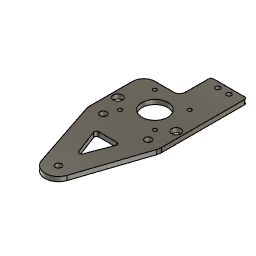
Laser Carriage - Motor Side V2 (Autodesk Fusion 360 design; units mm, degrees)
Autodesk Fusion 360 part; units mm, degrees
sketch "Sketch1" plane through (0, 0, 0) normal (0, 0, 1) x (1, 0, 0) in component "Laser Carriage - Motor Side V2"
  line L0 (0, 0) -> (64, 0)
  line L1 (64, 0) -> (64, 120)
  line L2 (64, 120) -> (0, 120)
  line L3 (0, 120) -> (0, 0)
  dimension "d1" = 64
  dimension "d2" = 120
  constraint horizontal L0
  constraint vertical L1
  constraint horizontal L2
  constraint vertical L3
  constraint coincident L0.start L3.end
  measures "d1" distance of L0.start L0.end
  measures "d2" distance of L0.start L2.end
extrude "Extrude1" add sketch "Sketch1" along normal blind 4 in component "Laser Carriage - Motor Side V2"
sketch "Sketch2" plane through (0, 0, 4) normal (0, 0, 1) x (-1, 0, 0) in component "Laser Carriage - Motor Side V2"
  line L0 (0, -120) -> (0, 0)
  line L1 (0, 0) -> (-64, 0)
  line L2 (-64, 0) -> (-64, -120)
  line L3 (-64, -120) -> (0, -120)
  line L4 (-12, -120) -> (-12, 0) construction
  line L5 (-52, -120) -> (-52, 0) construction
  line L6 (0, -12) -> (-64, -12) construction
  line L7 (0, -72) -> (-64, -72) construction
  circle A0 centre (-12, -72) radius 12 construction
  circle A1 centre (-52, -72) radius 12 construction
  circle A2 centre (-12, -72) radius 3
  circle A3 centre (-52, -72) radius 3
  circle A4 centre (-32, -12) radius 12 construction
  circle A5 centre (-32, -12) radius 2.75
  line L8 (0, -85) -> (-64, -85) construction
  line L9 (-32, -85) -> (-32, 0) construction
  line L10 (0, -42) -> (-64, -42) construction
  line L11 (0, -27) -> (-64, -27) construction
  line L12 (0, -56) -> (-64, -56) construction
  line L13 (-21, -56) -> (-21, -27) construction
  line L14 (-43, -56) -> (-43, -27) construction
  line L15 (-21, -56) -> (-43, -56)
  line L16 (-43, -56) -> (-32, -27)
  line L17 (-32, -27) -> (-21, -56)
  point P0 (-32, -42)
  dimension "d8" = 12
  dimension "d13" = 24
  dimension "d14" = 24
  dimension "d16" = 6
  dimension "d17" = 6
  dimension "d40" = 60
  dimension "d53" = 24
  dimension "d55" = 5.5
  dimension "d234" = 13
  dimension "d238" = 20
  dimension "d324" = 30
  dimension "d327" = 20
  dimension "d333" = 15
  dimension "d334" = 56
  dimension "d335" = 11
  dimension "d336" = 11
  constraint coincident L3 L4.start
  constraint coincident L1 L4.end
  constraint perpendicular L1 L4
  constraint coincident L3 L5.start
  constraint coincident L1 L5.end
  constraint perpendicular L1 L5
  constraint coincident L1 L9.end
  constraint coincident L0 L6.start
  constraint coincident L2 L6.end
  constraint perpendicular L2 L6
  constraint coincident L0 L7.start
  constraint coincident L2 L7.end
  constraint perpendicular L2 L7
  constraint coincident L7 A0.centre
  constraint coincident L4 A0.centre
  constraint coincident L7 A1.centre
  constraint coincident L5 A1.centre
  constraint concentric A0 A2
  constraint concentric A1 A3
  constraint coincident L6 A4.centre
  constraint concentric A4 A5
  constraint coincident L0 L8.start
  constraint coincident L2 L8.end
  constraint perpendicular L2 L8
  constraint midpoint L8 L9.start
  constraint coincident L0 L10.start
  constraint coincident L2 L10.end
  constraint perpendicular L2 L10
  constraint midpoint L10 P0
  constraint coincident A4.centre L9
  constraint coincident L0 L11.start
  constraint coincident L2 L11.end
  constraint perpendicular L2 L11
  constraint coincident L0 L12.start
  constraint coincident L2 L12.end
  constraint perpendicular L2 L12
  constraint coincident L12 L13.start
  constraint coincident L11 L13.end
  constraint perpendicular L11 L13
  constraint coincident L11 L14.end
  constraint perpendicular L11 L14
  constraint midpoint L11 L16.end
  constraint coincident L12 L14.start
  measures "d8" distance of L1 L6
  measures "d13" diameter of A0
  measures "d14" diameter of A1
  measures "d16" diameter of A2
  measures "d17" diameter of A3
  measures "d40" distance of L6 L7
  measures "d53" diameter of A4
  measures "d55" diameter of A5
  measures "d234" distance of A0.centre L8
  measures "d238" distance of L4 L9
  measures "d324" distance of L6 L10
  measures "d327" distance of L5 L9
  measures "d333" distance of L6 L11
  measures "d334" distance of L1 L12
  measures "d335" distance of L9 L13
  measures "d336" distance of L9 L14
extrude "Extrude2" cut sketch "Sketch2" against normal up to surface (4 mm away) contours A2 | A3 | A5 | L15 L16 L17 in component "Laser Carriage - Motor Side V2"
sketch "Sketch16" plane through (0, 0, 4) normal (0, 0, 1) x (-1, 0, 0) in component "Laser Carriage - Motor Side V2"
  circle A0 centre (-52, -72) radius 3
  circle A1 centre (-12, -72) radius 3
  line L0 (-64, -120) -> (0, -120)
  line L1 (0, -120) -> (0, 0)
  line L2 (0, 0) -> (-64, 0)
  line L3 (-64, 0) -> (-64, -120)
  circle A2 centre (-32, -12) radius 2.75
  line L4 (0, -91) -> (-64, -91) construction
  line L5 (-64, -120) -> (0, -120) construction
  line L6 (-6, 0) -> (-6, -120) construction
  line L7 (0, -120) -> (0, 0) construction
  line L8 (-58, 0) -> (-58, -120) construction
  circle A3 centre (-6, -91) radius 4
  circle A4 centre (-58, -91) radius 4
  line L9 (0, 0) -> (-64, 0)
  line L10 (-43, -56) -> (-32, -27)
  line L11 (-32, -27) -> (-21, -56)
  line L12 (-21, -56) -> (-43, -56)
  dimension "d268" = 6
  dimension "d269" = 6
  dimension "d270" = 8
  dimension "d271" = 8
  dimension "d273" = 91
  constraint coincident L1 L4.start
  constraint coincident L3 L4.end
  constraint perpendicular L3 L4
  constraint coincident L5 L6.end
  constraint coincident L2 L8.start
  constraint coincident L5 L8.end
  constraint coincident L4 A3.centre
  constraint coincident L6 A3.centre
  constraint coincident L4 A4.centre
  constraint coincident L8 A4.centre
  measures "d268" distance of L6 L7
  measures "d269" distance of L3 L8
  measures "d270" diameter of A3
  measures "d271" diameter of A4
  measures "d273" distance of L2 L4
extrude "Extrude17" cut sketch "Sketch16" against normal up to surface (4 mm away) contours A3 | A4 in component "Laser Carriage - Motor Side V2"
sketch "Sketch18" plane through (0, 0, 4) normal (0, 0, 1) x (-1, 0, 0) in component "Laser Carriage - Motor Side V2"
  line L0 (-64, -120) -> (0, -120)
  line L1 (-32, -120) -> (-32, 0) construction
  line L2 (0, 0) -> (-64, 0) construction
  line L3 (-47.5, -120) -> (-47.5, 0) construction
  line L4 (-16.5, 0) -> (-16.5, -120) construction
  line L5 (-2, -113.5) -> (-62, -113.5) construction
  line L6 (-2, -82.5) -> (-62, -82.5) construction
  line L7 (-2, -98) -> (-62, -98) construction
  circle A0 centre (-32, -98) radius 11.5
  circle A1 centre (-16.5, -113.5) radius 1.65
  circle A2 centre (-47.5, -113.5) radius 1.65
  circle A3 centre (-16.5, -82.5) radius 1.65
  circle A4 centre (-47.5, -82.5) radius 1.65
  line L8 (-2, -120) -> (-62, -120) construction
  line L9 (-54, -120) -> (-10, -120) construction
  line L10 (-10, -120) -> (-10, -76) construction
  line L11 (-10, -76) -> (-54, -76) construction
  line L12 (-54, -76) -> (-54, -120) construction
  line L13 (-54, -120) -> (-10, -76) construction
  line L14 (-10, -120) -> (-54, -76) construction
  point P0 (-32, -98)
  dimension "d275" = 15.5
  dimension "d276" = 15.5
  dimension "d279" = 98
  dimension "d280" = 15.5
  dimension "d281" = 15.5
  dimension "d283" = 23
  dimension "d284" = 3.3
  dimension "d285" = 3.3
  dimension "d286" = 3.3
  dimension "d287" = 3.3
  dimension "d288" = 6.5
  dimension "d289" = 44
  dimension "d290" = 44
  constraint midpoint L0 L1.start
  constraint perpendicular L0 L1
  constraint coincident L0 L3.start
  constraint coincident L2 L3.end
  constraint perpendicular L2 L3
  constraint coincident L2 L4.start
  constraint coincident L0 L4.end
  constraint perpendicular L0 L4
  constraint horizontal L5
  constraint horizontal L6
  constraint perpendicular L3 L7
  constraint midpoint L7 P0
  constraint coincident L4 A1.centre
  constraint coincident L5 A1.centre
  constraint coincident L3 A2.centre
  constraint coincident L5 A2.centre
  constraint coincident L4 A3.centre
  constraint coincident L6 A3.centre
  constraint coincident L3 A4.centre
  constraint coincident L6 A4.centre
  constraint perpendicular L3 L8
  constraint horizontal L9
  constraint perpendicular L9 L10
  constraint parallel L9 L11
  constraint parallel L10 L12
  constraint coincident L13 P0
  constraint coincident L14 P0
  constraint coincident P0 A0.centre
  measures "d275" distance of L1 L3
  measures "d276" distance of L1 L4
  measures "d279" distance of L2 L7
  measures "d280" distance of L5 L7
  measures "d281" distance of L6 L7
  measures "d283" diameter of A0
  measures "d284" diameter of A1
  measures "d285" diameter of A2
  measures "d286" diameter of A3
  measures "d287" diameter of A4
  measures "d288" distance of L5 L8
  measures "d289" distance of L10.end L11.end
  measures "d290" distance of L9.end L10.end
extrude "Extrude18" cut sketch "Sketch18" against normal up to surface (4 mm away) in component "Laser Carriage - Motor Side V2"
sketch "Sketch20" plane through (0, 0, 0) normal (0, 0, -1) x (1, 0, 0) in component "Laser Carriage - Motor Side V2"
  circle A0 centre (16.5, -113.5) radius 1.65
  circle A1 centre (47.5, -113.5) radius 1.65
  circle A2 centre (16.5, -82.5) radius 1.65
  circle A3 centre (32, -98) radius 11.5
  circle A4 centre (47.5, -82.5) radius 1.65
  circle A5 centre (6, -91) radius 4
  circle A6 centre (58, -91) radius 4
  circle A7 centre (52, -72) radius 3
  circle A8 centre (32, -12) radius 2.75
  circle A9 centre (12, -72) radius 3
  line L0 (0, 0) -> (0, -120)
  line L1 (0, -120) -> (64, -120)
  line L2 (64, -120) -> (64, 0)
  line L3 (64, 0) -> (0, 0)
  line L4 (64, -120) -> (64, -148)
  line L5 (32, -120) -> (32, -148)
  line L6 (32, -148) -> (64, -148)
  line L7 (32, -27) -> (43, -56)
  line L8 (43, -56) -> (21, -56)
  line L9 (21, -56) -> (32, -27)
  dimension "d303" = 28
  dimension "d304" = 28
  constraint coincident L1.end L2.start
  constraint perpendicular L1 L4
  constraint midpoint L1 L5.start
  constraint perpendicular L1 L5
  measures "d303" distance of L1.end L4.end
  measures "d304" distance of L5.start L5.end
extrude "Extrude20" add sketch "Sketch20" against normal blind 4 contours L1 L4 L5 L6 in component "Laser Carriage - Motor Side V2"
sketch "Sketch21" plane through (0, 0, 4) normal (0, 0, 1) x (-1, 0, 0) in component "Laser Carriage - Motor Side V2"
  circle A0 centre (-16.5, -113.5) radius 1.65
  circle A1 centre (-47.5, -113.5) radius 1.65
  circle A2 centre (-16.5, -82.5) radius 1.65
  circle A3 centre (-32, -98) radius 11.5
  circle A4 centre (-47.5, -82.5) radius 1.65
  circle A5 centre (-6, -91) radius 4
  circle A6 centre (-58, -91) radius 4
  line L0 (0, -120) -> (0, 0)
  line L1 (0, 0) -> (-64, 0)
  line L2 (-64, 0) -> (-64, -148)
  line L3 (-64, -148) -> (-32, -148)
  line L4 (-32, -148) -> (-32, -120)
  line L5 (-32, -120) -> (0, -120)
  circle A7 centre (-52, -72) radius 3
  circle A8 centre (-32, -12) radius 2.75
  circle A9 centre (-12, -72) radius 3
  line L6 (-48, -148) -> (-48, -122) construction
  line L7 (-32, -138) -> (-64, -138) construction
  line L8 (-54, -120) -> (-10, -120) construction
  line L9 (-32, -143) -> (-64, -143) construction
  line L10 (-53, -148) -> (-53, -138) construction
  line L11 (-43, -148) -> (-43, -138) construction
  circle A10 centre (-43, -143) radius 2.05
  circle A11 centre (-53, -143) radius 2.05
  line L12 (-43, -56) -> (-32, -27)
  line L13 (-32, -27) -> (-21, -56)
  line L14 (-21, -56) -> (-43, -56)
  dimension "d309" = 18
  dimension "d310" = 5
  dimension "d311" = 10
  dimension "d312" = 5
  dimension "d313" = 4.1
  dimension "d314" = 4.1
  constraint midpoint L3 L6.start
  constraint perpendicular L3 L6
  constraint coincident L4 L7.start
  constraint coincident L2 L7.end
  constraint perpendicular L2 L7
  constraint coincident L4 L9.start
  constraint coincident L2 L9.end
  constraint perpendicular L2 L9
  constraint coincident L3 L10.start
  constraint coincident L7 L10.end
  constraint perpendicular L7 L10
  constraint coincident L3 L11.start
  constraint coincident L7 L11.end
  constraint perpendicular L7 L11
  constraint midpoint L11 A10.centre
  constraint midpoint L10 A11.centre
  measures "d309" distance of L7 L8
  measures "d310" distance of L3 L9
  measures "d311" distance of L10 L11
  measures "d312" distance of L6 L11
  measures "d313" diameter of A10
  measures "d314" diameter of A11
extrude "Extrude21" cut sketch "Sketch21" against normal blind 4 contours A10 | A11 in component "Laser Carriage - Motor Side V2"
sketch "Sketch22" plane through (0, 0, 4) normal (0, 0, 1) x (-1, 0, 0) in component "Laser Carriage - Motor Side V2"
  circle A0 centre (-43, -143) radius 2.05
  circle A1 centre (-53, -143) radius 2.05
  circle A2 centre (-16.5, -113.5) radius 1.65
  circle A3 centre (-47.5, -113.5) radius 1.65
  circle A4 centre (-16.5, -82.5) radius 1.65
  circle A5 centre (-32, -98) radius 11.5
  circle A6 centre (-47.5, -82.5) radius 1.65
  circle A7 centre (-6, -91) radius 4
  circle A8 centre (-58, -91) radius 4
  circle A9 centre (-12, -72) radius 3
  circle A10 centre (-52, -72) radius 3
  circle A11 centre (-32, -12) radius 2.75
  line L0 (0, -120) -> (0, 0)
  line L1 (0, 0) -> (-64, 0)
  line L2 (-64, 0) -> (-64, -148)
  line L3 (-64, -148) -> (-32, -148)
  line L4 (-32, -148) -> (-32, -120)
  line L5 (-32, -120) -> (0, -120)
  circle A12 centre (-12, -72) radius 12
  circle A13 centre (-52, -72) radius 12
  circle A14 centre (-32, -12) radius 12
  line L6 (-0.6158, -68.2053) -> (-20.6158, -8.2053)
  line L7 (-63.3842, -68.2053) -> (-43.3842, -8.2053)
  line L8 (-43, -56) -> (-32, -27)
  line L9 (-32, -27) -> (-21, -56)
  line L10 (-21, -56) -> (-43, -56)
  dimension "d328" = 24
  dimension "d329" = 24
  dimension "d330" = 24
  constraint concentric A9 A12
  constraint concentric A10 A13
  constraint concentric A11 A14
  constraint tangent A12 L6
  constraint tangent A14 L6
  constraint tangent A13 L7
  constraint tangent A14 L7
  constraint coincident A13 L7.start
  constraint coincident A14 L7.end
  constraint coincident A14 L6.end
  constraint coincident A12 L6.start
  measures "d328" diameter of A12
  measures "d329" diameter of A13
  measures "d330" diameter of A14
extrude "Extrude22" cut sketch "Sketch22" against normal up to surface (4 mm away) contours L0 L1 A12 A14 L6 | L1 L2 A13 A14 L7 in component "Laser Carriage - Motor Side V2"
sketch "Sketch23" plane through (0, 0, 4) normal (0, 0, 1) x (-1, 0, 0) in component "Laser Carriage - Motor Side V2"
  arc A0 (-63.3842, -68.2053) -> (-64, -72) centre (-52, -72) ccw
  line L0 (-64, -72) -> (-64, -148)
  line L1 (-64, -148) -> (-32, -148)
  line L2 (-32, -148) -> (-32, -120)
  line L3 (-32, -120) -> (0, -120)
  line L4 (0, -120) -> (0, -72)
  arc A1 (0, -72) -> (-0.6158, -68.2053) centre (-12, -72) ccw
  line L5 (-0.6158, -68.2053) -> (-20.6158, -8.2053)
  arc A2 (-20.6158, -8.2053) -> (-43.3842, -8.2053) centre (-32, -12) ccw
  line L6 (-43.3842, -8.2053) -> (-63.3842, -68.2053)
  circle A3 centre (-43, -143) radius 2.05
  circle A4 centre (-53, -143) radius 2.05
  circle A5 centre (-16.5, -113.5) radius 1.65
  circle A6 centre (-47.5, -113.5) radius 1.65
  circle A7 centre (-16.5, -82.5) radius 1.65
  circle A8 centre (-32, -98) radius 11.5
  circle A9 centre (-47.5, -82.5) radius 1.65
  circle A10 centre (-6, -91) radius 4
  circle A11 centre (-58, -91) radius 4
  circle A12 centre (-12, -72) radius 3
  circle A13 centre (-52, -72) radius 3
  circle A14 centre (-32, -12) radius 2.75
  line L7 (-43, -56) -> (-32, -27)
  line L8 (-32, -27) -> (-21, -56)
  line L9 (-21, -56) -> (-43, -56)
fillet "Fillet11" radius 5 1 edges at (32, 120, 2) in component "Laser Carriage - Motor Side V2"
fillet "Fillet11" radius 2 2 edges at (32, 148, 2) (64, 148, 2) in component "Laser Carriage - Motor Side V2"
fillet "Fillet11" radius 2 3 edges at (21, 56, 2) (43, 56, 2) (32, 27, 2) in component "Laser Carriage - Motor Side V2"
fillet "Fillet11" radius 10 1 edges at (0, 120, 2) in component "Laser Carriage - Motor Side V2"
component "Laser Carriage - Motor Side V2" placed x (1, 0, 0) y (0, 1, 0) z (0, 0, 1) at (0, 0, 0)
named bodies: "Laser Carriage - Motor Side V2"
